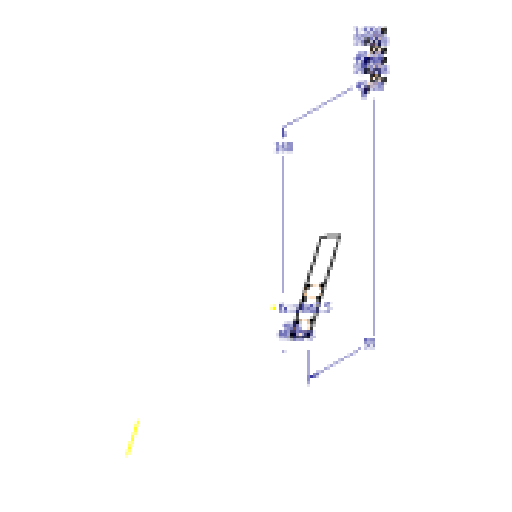
# Autodesk Inventor part: OutakeSlidePlate
Saved by Autodesk Inventor 2023 (Build 270158000, 158)
## iProperties
Created: 2022-11-09
Part Number: OutakeSlidePlate
Material: Generic
Document SubType Name: Modeling
Designer: deli
Density: 1 g/cm^3
Appearance: Default
Author: deli
Autodesk Inventor part; units mm, degrees
ref_plane "YZ Plane" through (0, 0, 0) normal (1, 0, 0) x (0, 1, 0)
ref_plane "XZ Plane" through (0, 0, 0) normal (0, 1, 0) x (-1, 0, 0)
ref_plane "XY Plane" through (0, 0, 0) normal (0, 0, 1) x (1, 0, 0)
sketch "Sketch1" plane through (0, 0, 0) normal (1, 0, 0) x (0, 1, 0)
  circle A0 centre (-75.2256, -24.4411) radius 1.1
  circle A1 centre (-79.9605, -35.4675) radius 1.1
  circle A2 centre (-67.8747, -27.5977) radius 1.1
  circle A3 centre (-72.6096, -38.6241) radius 1.1
  circle A4 centre (-54.5512, -33.319) radius 1.1
  circle A5 centre (-59.286, -44.3454) radius 1.1
  circle A6 centre (-47.2003, -36.4756) radius 1.1
  circle A7 centre (-51.9351, -47.502) radius 1.1
  line L0 (-75.2256, -24.4411) -> (-67.8747, -27.5977) construction
  line L1 (-67.8747, -27.5977) -> (-72.6096, -38.6241) construction
  line L2 (-72.6096, -38.6241) -> (-79.9605, -35.4675) construction
  line L3 (-79.9605, -35.4675) -> (-75.2256, -24.4411) construction
  line L4 (-54.5512, -33.319) -> (-47.2003, -36.4756) construction
  line L5 (-47.2003, -36.4756) -> (-51.9351, -47.502) construction
  line L6 (-51.9351, -47.502) -> (-59.286, -44.3454) construction
  line L7 (-59.286, -44.3454) -> (-54.5512, -33.319) construction
  line L8 (-76.7661, -21.0589) -> (-84.7483, -39.6475)
  line L9 (169.6149, -96.3481) -> (190.2893, -105.226) projected
  circle A8 centre (-74.4613, -97.502) radius 4
  circle A9 centre (-67.5465, -90.5872) radius 1.778
  circle A10 centre (-67.5465, -104.4168) radius 1.778
  circle A11 centre (-81.3761, -104.4168) radius 1.778
  circle A12 centre (-81.3761, -90.5872) radius 1.778
  line L10 (-67.5465, -90.5872) -> (-81.3761, -104.4168) construction
  line L11 (-67.5465, -104.4168) -> (-81.3761, -90.5872) construction
  line L12 (-81.3761, -90.5872) -> (-81.3761, -104.4168) construction
  line L13 (-67.5465, -90.5872) -> (-67.5465, -104.4168) construction
  circle A13 centre (-53.8873, -97.502) radius 4
  circle A14 centre (-46.9725, -90.5872) radius 1.778
  circle A15 centre (-46.9725, -104.4168) radius 1.778
  circle A16 centre (-60.8021, -104.4168) radius 1.778
  circle A17 centre (-60.8021, -90.5872) radius 1.778
  line L14 (-46.9725, -90.5872) -> (-60.8021, -104.4168) construction
  line L15 (-46.9725, -104.4168) -> (-60.8021, -90.5872) construction
  line L16 (-60.8021, -90.5872) -> (-60.8021, -104.4168) construction
  line L17 (-46.9725, -90.5872) -> (-46.9725, -104.4168) construction
  line L18 (-81.3761, -107.789) -> (-46.9725, -107.789)
  line L19 (-43.6003, -104.4168) -> (-43.6003, -36.4756)
  arc A18 (-46.9725, -107.789) -> (-43.6003, -104.4168) centre (-46.9725, -104.4168) ccw
  line L20 (-53.8873, -97.502) -> (-74.4613, -97.502) construction
  arc A19 (-84.7483, -104.4168) -> (-81.3761, -107.789) centre (-81.3761, -104.4168) ccw
  line L21 (-76.7661, -21.0589) -> (-45.8901, -33.1224)
  arc A20 (-43.6003, -36.4756) -> (-45.8901, -33.1224) centre (-47.2003, -36.4756) ccw
  line L22 (-84.7483, -104.4168) -> (-84.7483, -39.6475)
  point P0 (0, 0)
  dimension "d0" = 2.2
  dimension "d1" = 12
  dimension "d2" = 8
  dimension "d3" = 14.5
  dimension "d7" = 2.75
  dimension "d8" = 8
  dimension "d12" = 3.556
  dimension "d13" = 19.558
  dimension "d14" = 45
  dimension "d16" = 8
  dimension "d17" = 3.556
  dimension "d18" = 19.558
  dimension "d19" = 45
  dimension "d20" = 20.574
  dimension "d26" = 3.3722
  dimension "d27" = 13.8296
  dimension "d30" = 2.5
  dimension "d33" = 2.5
  dimension "d34" = 50
  constraints: 45 end point, 21 centre point, 14 equal radius, 9 perpendicular, 7 point on circle, 6 equal length, 6 tangent, 4 coincident, 4 midpoint, 4 vertical, 1 collinear, 1 concentric, 1 horizontal, 1 parallel, 1 point on line
  measures "d0" diameter of A0
  measures "d1" distance of L2.end L0.start
  measures "d2" distance of L0.start L0.end
  measures "d3" distance between parallel lines of L7 L1
  measures "d7" distance between parallel lines of L3 L8
  measures "d8" diameter of A8
  measures "d12" diameter of A9
  measures "d13" distance of L10.start L10.end
  measures "d14" angle of L12 L11
  measures "d16" diameter of A13
  measures "d17" diameter of A14
  measures "d18" distance of L14.start L16.end
  measures "d19" angle of L16 L15
  measures "d20" distance of A13.centre A8.centre
  measures "d26" radius of A18
  measures "d27" distance of L14.start L15.start
  measures "d30" distance from line of L0 L8.start
  measures "d33" radial gap between concentric circles of A6 A20
  measures "d34" vertical distance of A8.centre L5.end
extrude "Extrusion1" add sketch "Sketch1" along normal blind 3.175
equation "\"d33\" = d30"
body "Solid1"
